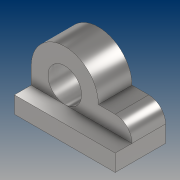
# Autodesk Inventor part: 4
Saved by Autodesk Inventor 2020.2 (Build 242310000, 310)
## iProperties
Created: 2020-09-17
Part Number: 4
Material: 鋼、碳鋼
Document SubType Name: Modeling
Designer: user
Density: 7.85 g/cm^3
Appearance: 半拋光
Mass: 281.454 g
Surface Area: 92.1283 cm^2
Volume: 35.854 cm^3
Author: user
Autodesk Inventor part; units mm, degrees
ref_plane "YZ Plane" through (0, 0, 0) normal (1, 0, 0) x (0, 1, 0)
ref_plane "XZ Plane" through (0, 0, 0) normal (0, 1, 0) x (-1, 0, 0)
ref_plane "XY Plane" through (0, 0, 0) normal (0, 0, 1) x (1, 0, 0)
sketch "草圖1" plane through (0, 0, 0) normal (0, 0, 1) x (1, 0, 0)
  line L0 (0, 0) -> (0, 20)
  arc A0 (40, 20) -> (0, 20) centre (20, 20) ccw
  line L1 (40, 20) -> (50, 20)
  arc A1 (60, 10) -> (50, 20) centre (50, 10) ccw
  line L2 (60, 10) -> (60, 0)
  line L3 (60, 0) -> (0, 0)
  dimension "d0" = 20
  dimension "d1" = 10
  dimension "d2" = 60
  dimension "d3" = 20
  dimension "d4" = 20
  constraints: 8 end point, 4 point on circle, 3 perpendicular, 3 tangent, 2 centre point, 1 vertical
  measures "d0" distance of L0.start L0.end
  measures "d1" distance of L2.start L2.end
  measures "d2" distance of L2.end L0.start
  measures "d3" distance from line of A0.centre L0
  measures "d4" distance between parallel lines of L3 L1
extrude "擠出1" add sketch "草圖1" along normal blind 30
sketch "草圖2" plane through (0, 0, 0) normal (1, 0, 0) x (0, 1, 0)
  line L0 (49.6767, 20) -> (10, 20)
  line L1 (10, 20) -> (10, 40.4278)
  line L2 (10, 40.4278) -> (49.6767, 40.4278)
  line L3 (49.6767, 40.4278) -> (49.6767, 20)
  line L4 (0, 0) -> (0, 30) projected
  line L5 (20, 30) -> (0, 30) projected
  dimension "d7" = 10
  dimension "d8" = 10
  constraints: 8 end point, 2 parallel, 1 horizontal, 1 perpendicular
  measures "d7" distance between parallel lines of L1 L4
  measures "d8" distance between parallel lines of L0 L5
extrude "擠出2" cut sketch "草圖2" along normal blind 74.5
sketch "草圖3" plane through (20, 20, 20) normal (0, 0, 1) x (1, 0, 0)
  line L0 (-20, -10) -> (40, -10) projected
  arc A0 (40, -10) -> (30, 0) centre (30, -10) ccw projected
  line L1 (20, 0) -> (30, 0) projected
  arc A1 (20, 0) -> (-20, 0) centre (0, 0) ccw projected
  line L2 (-20, -10) -> (-20, 0) projected
  line L3 (-20, -20) -> (-20, -10) projected
  line L4 (40, -20) -> (-20, -20) projected
  line L5 (40, -10) -> (40, -20) projected
  circle A2 centre (0, 0) radius 10
  dimension "d11" = 20
  constraints: 1 centre point, 1 coincident
  measures "d11" diameter of A2
extrude "擠出3" cut sketch "草圖3" against normal through all contours A2
